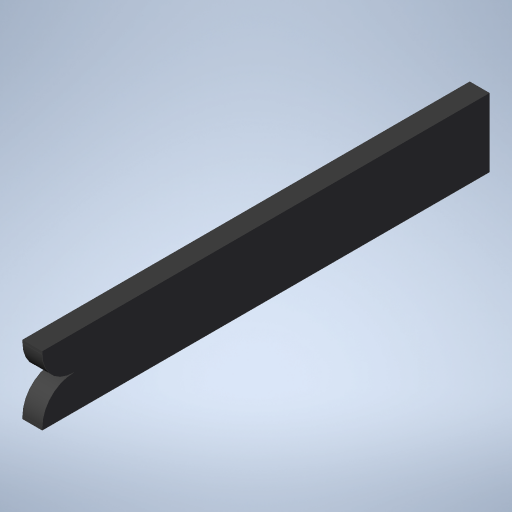
# Autodesk Inventor part: Part2
Saved by Autodesk Inventor 2024 (Build 280153000, 153)
## iProperties
Created: 2024-06-12
Part Number: Part2
Material: Generic
Document SubType Name: Modeling
Designer: albah
Density: 1 g/cm^3
Appearance: Default
Author: albah
Autodesk Inventor part; units mm, degrees
ref_plane "YZ Plane" through (0, 0, 0) normal (1, 0, 0) x (0, 1, 0)
ref_plane "XZ Plane" through (0, 0, 0) normal (0, 1, 0) x (-1, 0, 0)
ref_plane "XY Plane" through (0, 0, 0) normal (0, 0, 1) x (1, 0, 0)
sketch "Sketch1" plane through (0, 0, 0) normal (0, 0, 1) x (1, 0, 0)
  line L0 (0, 0) -> (10, 0)
  line L1 (10, 0) -> (10, 35)
  line L2 (10, 35) -> (0, 35)
  line L3 (0, 35) -> (0, 0)
  dimension "d0" = 10
  dimension "d1" = 35
  constraints: 8 end point, 2 parallel, 1 horizontal, 1 perpendicular
  measures "d0" distance of L2.end L1.end
  measures "d1" distance of L1.end L0.end
extrude "Extrusion1" add sketch "Sketch1" along normal blind 160
sketch "Sketch2" plane through (0, 0, 160) normal (0, 0, 1) x (1, 0, 0)
  line L0 (0, 35) -> (0, 0) projected
  line L1 (0, 17.5) -> (10, 17.5)
  line L2 (10, 0) -> (10, 35) projected
  line L3 (0, 35) -> (10, 35)
  line L4 (0, 0) -> (10, 0)
  constraints: 6 end point, 2 midpoint, 1 parallel, 1 perpendicular
extrude "Extrusion2" add sketch "Sketch2" along normal blind 68 contours L1 L2 L4 L0
fillet "Fillet1" radius 16 1 edges at (5, 17.5, 228)
sketch "Sketch4" plane through (0, 0, 160) normal (0, 0, 1) x (1, 0, 0)
  point P0 (0, 0)
move faces "Move1" translate (0, 0, 68) faces at (3.3333, 23.3333, 160)
fillet "Fillet2" radius 16 1 edges at (5, 17.5, 228)
equation "\"BendRadius\" = Thickness"
equation "\"BendReliefWidth\" = Thickness"
equation "\"BendReliefDepth\" = 0.5 * Thickness"
equation "\"CornerReliefSize\" = 4 * Thickness"
equation "\"MinimumRemnant\" = 2 * Thickness"
equation "\"TransitionRadius\" = BendRadius"
equation "\"JacobiRadiusSize\" = BendRadius"
equation "\"GapSize\" = Thickness"
equation "\"Thickness\" = 0.5"
body "Solid1"
